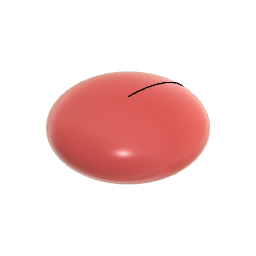
red_smartie (Autodesk Fusion 360 design; units mm, degrees)
Autodesk Fusion 360 part; units mm, degrees
note: some values were not read from the file. Set by a fixed rule: which sketch regions a step uses.
sketch "Smartie Outline" plane through (0, 0, 0) normal (1, 0, 0) x (0, 1, 0)
  spline S0 degree 5 poles (-7.5, 0) (-7.5, 0.2185) (-7.4248, 0.6556) (-7.0865, 1.3008) (-6.2029, 2.0984) (-4.4965, 2.8947) (-2.3601, 3.4101) (0, 3.5892) (2.3601, 3.4101) (4.4965, 2.8947) (6.2029, 2.0984) (7.3074, 1.1014) (7.6911, 0) (7.3074, -1.1014) (6.2029, -2.0984) (4.4965, -2.8947) (2.3601, -3.4101) (0, -3.5892) (-2.3601, -3.4101) (-4.4965, -2.8947) (-6.2029, -2.0984) (-7.0865, -1.3008) (-7.4248, -0.6556) (-7.5, -0.2185) (-7.5, 0) knots 0 0 0 0 0 0 0.05 0.1 0.15 0.2 0.25 0.3 0.35 0.4 0.45 0.5 0.55 0.6 0.65 0.7 0.75 0.8 0.85 0.9 0.95 1 1 1 1 1 1
  line L0 (0, -3.5) -> (0, 3.5)
  point P0 (0, 3.5)
  point P1 (7.5, 0)
  point P2 (0, -3.5)
  dimension "d3" = 3.5
  dimension "d4" = 3.5
  dimension "d5" = 7.5
  dimension "d6" = 7.5
  constraint coincident P2 L0.start
  constraint coincident P0 L0.end
  constraint vertical L0
  measures "d3" distance of origin L0.end
  measures "d4" distance of origin P2
  measures "d5" distance of origin S0.start
  measures "d6" distance of origin P1
revolve "Revolve1" add sketch "Smartie Outline" angle 360 about axis through (0, 0, -3.5) along (0, 0, 1) contours S0 L0 picked at (-1.0058, -1.1492)
equation "smartieWidth = 15 mm" comment "Major axis of the Smartie"
equation "smartieHeight = 7 mm" comment "Minor axis of the Smartie"
equation "d3 = smartieHeight / 2"
equation "d4 = smartieHeight / 2"
equation "d5 = smartieWidth / 2"
equation "d6 = smartieWidth / 2"
named bodies: "Red Smartie"
